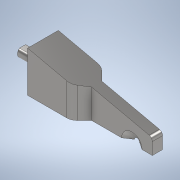
# Autodesk Inventor part: blade
Saved by Autodesk Inventor 2020 (Build 240168000, 168)
## iProperties
Created: 2019-12-24
Part Number: blade
Material: Stainless Steel
Document SubType Name: Modeling
Designer: metal
Density: 8 g/cm^3
Appearance: Semi-Polished
Mass: 3.38507 g
Surface Area: 5.45108 cm^2
Volume: 0.423134 cm^3
Author: metal
Autodesk Inventor part; units mm, degrees
ref_plane "YZ Plane" through (0, 0, 0) normal (1, 0, 0) x (0, 1, 0)
ref_plane "XZ Plane" through (0, 0, 0) normal (0, 1, 0) x (-1, 0, 0)
ref_plane "XY Plane" through (0, 0, 0) normal (0, 0, 1) x (1, 0, 0)
sketch "Sketch1" plane through (0, 0, 0) normal (0, 0, 1) x (1, 0, 0)
  line L0 (0, 8) -> (22.3923, 3)
  line L1 (22.3923, 0) -> (22.3923, 3)
  line L2 (0, 0) -> (22.3923, 0)
  line L3 (0, 8) -> (0, 0)
  dimension "d5" = 3
  dimension "d7" = 8
  dimension "d59" = 22.3923
  constraints: 8 end point, 2 vertical, 1 horizontal
  measures "d5" distance of L1.start L0.end
  measures "d7" distance of L0.start L2.start
  measures "d59" distance of L2.start L1.start
extrude "Extrusion1" add sketch "Sketch1" along normal mid plane 6
sketch "Sketch2" plane through (0, 0, 3) normal (-1, 0, 0) x (0, 0, 1)
  line L0 (-6, 0) -> (-6, 8) projected
  line L1 (0, 3) -> (0, 8) projected
  line L2 (-6, 0) -> (0, 8)
  line L3 (-6, 8) -> (0, 8) projected
  line L4 (0, 8) -> (0, 0) projected
  line L5 (-6, 8) -> (0, 0)
  arc A0 (-3.995, 3.9001) -> (-2.005, 3.9001) centre (-3, 4) ccw
  line L6 (-3.6, 4.8) -> (-2.4, 4.8)
  arc A1 (-2.005, 3.9001) -> (-2.4, 4.8) centre (-3, 4) ccw
  arc A2 (-3.6, 4.8) -> (-3.9949, 3.8993) centre (-3, 4) ccw
  point P0 (-3, 0)
  constraints: 6 end point, 6 point on circle, 3 centre point, 2 point on line, 1 midpoint
extrude "Extrusion2" add sketch "Sketch2" along normal blind 4 contours A0 A2 L5 L2 | L2 L5 A0 | L6 L2 L5 | L2 A1 A0 L5
sketch "Sketch3" plane through (0, 0, 3) normal (0, -1, 0) x (1, 0, 0)
  line L0 (22.3923, -6) -> (0, -6) projected
  line L1 (8.5053, -6) -> (10.5053, -4)
  line L2 (10.5053, -4) -> (22.3923, -4)
  line L3 (22.3923, 0) -> (22.3923, -6) projected
  line L4 (22.3923, -4) -> (22.3923, -6)
  line L5 (22.3923, -6) -> (8.5053, -6)
  line L6 (8.5053, 0) -> (10.5053, -2)
  line L7 (10.5053, -2) -> (22.3923, -2)
  line L8 (22.3923, -2) -> (22.3923, 5.9236)
  line L9 (22.3923, 0) -> (0, 0) projected
  line L10 (8.5053, 0) -> (22.3923, 0)
  point P0 (0, -3)
  dimension "d13" = 2
  dimension "d14" = 2
  dimension "d15" = 45
  constraints: 16 end point, 3 point on line, 2 collinear, 2 parallel, 2 perpendicular, 1 vertical alignment
  measures "d13" distance between parallel lines of L7 L2
  measures "d14" distance between parallel lines of L0 L2
  measures "d15" angle of L9 L6
extrude "Extrusion3" cut sketch "Sketch3" against normal through all
ref_plane "Work Plane2" through (15.7073, 3, 0) normal (-1, 0, 0) x (0, 0, -1)
ref_plane "Work Plane1" through (22.3923, 3, 0) normal (-1, 0, 0) x (0, 0, -1)
fillet "Fillet8" radius 2 1 edges at (8.5053, 3.0504, 3)
fillet "Fillet9" radius 2 1 edges at (8.5053, 3.0504, -3)
fillet "Fillet11" radius 0.8 1 edges at (22.3923, 3, 0)
sketch "Sketch13" plane through (10.5053, 0, 1) normal (0, 0, 1) x (1, 0, 0)
  line L0 (0, 0) -> (11.887, 0) projected
  arc A0 (9.887, 0) -> (5.887, 0) centre (7.887, 0) ccw
  point P0 (-10.5053, 0)
  dimension "d86" = 4
  dimension "d88" = 4
  constraints: 3 point on line, 2 point on circle, 1 centre point
  measures "d86" diameter of A0
  measures "d88" distance of L0.end A0.centre
ref_plane "Work Plane5" through (10.5053, 0, 0) normal (0, 0, 1) x (1, 0, 0)
sketch "Sketch14" plane through (10.5053, 0, 0) normal (0, 0, 1) x (1, 0, 0)
  line L0 (0, 0) -> (11.887, 0) projected
  arc A0 (8.387, 0) -> (7.387, 0) centre (7.887, 0) ccw
  point P0 (-10.5053, 0)
  dimension "d89" = 4
  dimension "d90" = 1
  constraints: 3 point on line, 2 point on circle, 1 centre point
  measures "d89" distance of L0.end A0.centre
  measures "d90" diameter of A0
loft "Loft1" cut profiles "Sketch13", "Sketch14"
sketch "Sketch16" plane through (22.3923, 0, -1) normal (0, 0, -1) x (-1, 0, 0)
  arc A0 (6, 0) -> (2, 0) centre (4, 0) ccw
  line L0 (0, 0) -> (2, 0) projected
  line L1 (6, 0) -> (11.887, 0) projected
  line L2 (2, 0) -> (6, 0)
  line L3 (11.887, 0) -> (0, 0) projected
  point P0 (22.3923, 0)
  dimension "d98" = 4
  dimension "d99" = 4
  constraints: 3 end point, 2 point on circle, 1 centre point, 1 collinear
  measures "d98" diameter of A0
  measures "d99" distance of L0.start A0.centre
sketch "Sketch17" plane through (10.5053, 0, 0) normal (0, 0, 1) x (1, 0, 0)
  line L0 (11.887, 2.3589) -> (11.887, 0) projected
  line L1 (9.887, 0) -> (8.387, 0) projected
  line L2 (8.8124, 0) -> (7.1201, 0)
  arc A0 (8.387, 0) -> (7.387, 0) centre (7.887, 0) ccw
  point P0 (-10.5053, 0)
  dimension "d102" = 4
  dimension "d103" = 1
  constraints: 4 point on line, 2 end point, 2 point on circle, 1 centre point, 1 collinear
  measures "d102" distance of L0.end A0.centre
  measures "d103" diameter of A0
loft "Loft2" cut profiles "Sketch16" section 2 edges at (18.3923, 0.5, 0) (18.3923, 0, 0)
body "Solid1"
